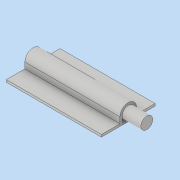
# Autodesk Inventor part: lw_5
Saved by Autodesk Inventor 2019 (Build 230136000, 136)
## iProperties
Created: 2021-04-29
Part Number: lw_5
Material: Типовые
Document SubType Name: Modeling
Designer: Kurbatova
Density: 1 g/cm^3
Appearance: По умолчанию
Author: Kurbatova
Autodesk Inventor part; units mm, degrees
ref_plane "YZ Plane" through (0, 0, 0) normal (1, 0, 0) x (0, 1, 0)
ref_plane "XZ Plane" through (0, 0, 0) normal (0, 1, 0) x (-1, 0, 0)
ref_plane "XY Plane" through (0, 0, 0) normal (0, 0, 1) x (1, 0, 0)
sketch "Цилиндр" plane through (0, 0, 0) normal (1, 0, 0) x (0, 1, 0)
  line L0 (5, 0) -> (-5, 0)
  line L1 (0, 5) -> (0, -5)
  circle A0 centre (0, 0) radius 5
  dimension "d0" = 10
  constraints: 4 end point, 4 point on circle, 2 midpoint, 1 centre point, 1 coincident, 1 horizontal, 1 vertical
  measures "d0" diameter of A0
extrude "Выдавливание1" add sketch "Цилиндр" along normal blind 80 and the other way blind 15.61
sketch "Корпус" plane through (-15.61, 0, 0) normal (-1, 0, 0) x (0, 0, 1)
  arc A0 (5, 0) -> (-5, 0) centre (0, 0) ccw
  circle A1 centre (0, 0) radius 5
  line L0 (0, 5) -> (0, -5)
  line L1 (-5, 0) -> (5, 0)
  line L2 (-4.999794, -5) -> (5, -5)
  arc A2 (5, 0) -> (-5, 0) centre (0, 0) ccw
  line L3 (5, 0) -> (4.993827, -5)
  line L4 (-4.993645, -5) -> (-5, 0)
  line L5 (-22.603669, -4.981004) -> (-22.603669, -6.955879)
  arc A3 (0, 7) -> (-7, -0.000001) centre (0, 0) ccw
  line L6 (-22.603669, -6.955879) -> (2.271039, -6.955879)
  line L7 (22.603669, -4.981004) -> (22.603669, -6.955879)
  arc A4 (7, -0.000001) -> (0, 7) centre (0, 0) ccw
  line L8 (22.603669, -6.955879) -> (2.271039, -6.955879)
  line L9 (-6.993669, -4.981004) -> (-7, -0.000001)
  line L10 (-22.603669, -4.981004) -> (-6.993669, -4.981004)
  line L11 (7, -0.000001) -> (6.99385, -4.981004)
  line L12 (22.603669, -4.981004) -> (6.99385, -4.981004)
  dimension "d12" = 15.61
  constraints: 26 end point, 12 point on circle, 5 horizontal, 4 centre point, 4 point on line, 3 symmetric about line, 2 midpoint, 2 parallel, 2 vertical, 1 coincident, 1 tangent, 1 other
  measures "d12" distance of L5.start L9.start
sketch "Корпус outline for Выдавливание2" plane through (-15.61, 0, 0) normal (-1, 0, 0) x (0, 0, 1)
  line L0 (-22.603669, -6.955879) -> (-22.603669, -4.981004)
  line L1 (2.271039, -6.955879) -> (-22.603669, -6.955879)
  line L2 (-22.603669, -4.981004) -> (-6.993669, -4.981004)
  line L3 (22.603669, -6.955879) -> (2.271039, -6.955879)
  line L4 (-6.993669, -4.981004) -> (-7, -0.000001)
  line L5 (22.603669, -4.981004) -> (22.603669, -6.955879)
  arc A0 (-7, -0.000001) -> (0, 7) centre (0, 0) cw
  line L6 (6.99385, -4.981004) -> (22.603669, -4.981004)
  arc A1 (0, 7) -> (7, -0.000001) centre (0, 0) cw
  line L7 (7, -0.000001) -> (6.99385, -4.981004)
  arc A2 (5, 0) -> (0, 5) centre (0, 0) ccw
  arc A3 (0, 5) -> (-5, 0) centre (0, 0) ccw
  line L8 (-5, 0) -> (-4.993645, -5)
  line L9 (-4.993645, -5) -> (0, -5)
  line L10 (0, -5) -> (4.993827, -5)
  line L11 (4.993827, -5) -> (5, 0)
extrude "Выдавливание2" add sketch "Корпус outline for Выдавливание2" against normal blind 80
sketch "Выемка" plane through (64.39, -0.000001, -7) normal (0, -0.001271, -0.9999992) x (-1, 0, 0)
  line L0 (80, -4.981007) -> (80, 0)
  line L1 (80, 0) -> (0, 0)
  line L2 (0, -4.981007) -> (0, 0)
  line L3 (80, -4.981007) -> (0, -4.981007)
  line L4 (80, -5.008896) -> (-15.61, -5.008896)
  line L5 (80, 6.991104) -> (0, 6.991104)
  line L6 (33.204769, 6.991104) -> (33.204769, -5.008896)
  line L7 (33.204769, 6.991104) -> (73.204769, 6.991104)
  line L8 (73.204769, -5.008896) -> (73.204769, 6.991104)
  line L9 (33.204769, -5.008896) -> (73.204769, -5.008896)
  line L10 (38.204769, 1.959942) -> (38.204769, -5.008896)
  line L11 (68.204769, 1.959942) -> (68.204769, -5.008896)
  line L12 (38.204769, -5.008896) -> (38.204769, 1.959942)
  line L13 (68.204769, 1.959942) -> (38.204769, 1.959942)
  line L14 (33.204769, -5.008896) -> (38.204769, -5.008896)
  line L15 (68.204769, -5.008896) -> (73.204769, -5.008896)
  point P0 (64.39, -0.008896)
  dimension "d15" = 30
  dimension "d22" = 5
  dimension "d23" = 5
  constraints: 20 end point, 6 point on line, 5 perpendicular, 3 parallel, 1 collinear, 1 vertical
  measures "d15" distance between parallel lines of L11 L10
  measures "d22" distance between parallel lines of L10 L6
  measures "d23" distance between parallel lines of L8 L11
extrude "Выдавливание3" cut sketch "Выемка" against normal blind 2 contours L8 L4 L11 L3 | L3 L11 L1 L8 | L1 L11 L13 L10 L6 L5 L8 | L10 L4 L6 L3 | L3 L6 L1 L10
